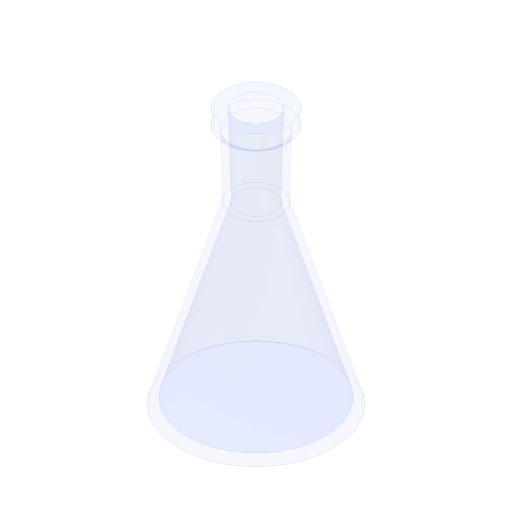
# Autodesk Inventor part: Модель колба коническая 25мл
Saved by Autodesk Inventor 2023 (Build 270158000, 158)
## iProperties
Created: 2022-06-09
Part Number: Модель колба коническая 25мл
Material: Типовые
Document SubType Name: Modeling
Designer: Admin
Density: 1 g/cm^3
Appearance: Вода — пузырьки
Author: Admin
Autodesk Inventor part; units mm, degrees
ref_plane "YZ Plane" through (0, 0, 0) normal (1, 0, 0) x (0, 1, 0)
ref_plane "XZ Plane" through (0, 0, 0) normal (0, 1, 0) x (-1, 0, 0)
ref_plane "XY Plane" through (0, 0, 0) normal (0, 0, 1) x (1, 0, 0)
sketch "Эскиз1" plane through (0, 0, 0) normal (0, 0, 1) x (1, 0, 0)
  line L0 (0, 0) -> (25.5, 0)
  line L1 (25.5, 0) -> (8, 58)
  line L2 (8, 58) -> (8.4582, 79)
  line L3 (10.5, 80) -> (10.5, 85)
  line L4 (10.5, 85) -> (6.5, 85)
  line L5 (6.5, 85) -> (5.9109, 58)
  line L6 (5.9109, 58) -> (22.8075, 2)
  line L7 (22.8075, 2) -> (0, 2)
  line L8 (0, 21.2466) -> (0, -2.9394)
  line L9 (8.4582, 79) -> (10.5, 80)
  line L10 (0, 0) -> (-25.5, 0)
  line L11 (-25.5, 0) -> (-8, 58)
  line L12 (-8, 58) -> (-8.4582, 79)
  line L13 (-10.5, 80) -> (-10.5, 85)
  line L14 (-10.5, 85) -> (-6.5, 85)
  line L15 (-6.5, 85) -> (-5.9109, 58)
  line L16 (-5.9109, 58) -> (-22.8075, 2)
  line L17 (-22.8075, 2) -> (0, 2)
  line L18 (-8.4582, 79) -> (-10.5, 80)
  line L19 (43.1283, 50) -> (10.4138, 50)
  line L20 (10.4138, 50) -> (8.3785, 49.8219)
  line L21 (-9.1205, 47.3626) -> (-11.1664, 47.5057)
  line L22 (-11.1664, 47.5057) -> (-43.7017, 44.0861)
  line L23 (25.1983, 1) -> (-25.1983, 1)
  line L24 (43.1283, -5) -> (-43.7017, -5)
  line L25 (-9.1205, 47.3626) -> (8.3785, 49.8219)
  point P0 (0, 2)
  dimension "d0" = 51
  dimension "d1" = 2
  dimension "d2" = 2
  dimension "d3" = 58
  dimension "d4" = 85
  dimension "d5" = 5
  dimension "d6" = 16
  dimension "d8" = 21
  dimension "d9" = 4
  dimension "d10" = 21
  dimension "d12" = 50
  dimension "d27" = 5
  dimension "d51" = 5
  dimension "d53" = 3
  dimension "d55" = 12
  dimension "d57" = 10
  dimension "d78" = 86.83
  constraints: 52 end point, 8 symmetric about line, 6 point on line, 4 parallel, 3 horizontal, 3 vertical alignment, 1 equal length, 1 horizontal alignment, 1 perpendicular, 1 vertical, 1 other
  measures "d0" diameter of L0.end L8
  measures "d1" distance between parallel lines of L7 L0
  measures "d2" distance between parallel lines of L1 L6
  measures "d3" vertical distance of L1.end L0.end
  measures "d4" distance between parallel lines of L4 L0
  measures "d5" distance of L3.start L3.end
  measures "d6" diameter of L1.end L8
  measures "d8" diameter of L3 L8
  measures "d9" distance of L3.end L4.end
  measures "d10" vertical distance of L2.end L1.end
  measures "d12" distance between parallel lines of L19 L0
  measures "d27" distance between parallel lines of L0 L24
  measures "d51" angle of L19 L20
  measures "d53" angle of L25 L20
  measures "d55" angle of L25 L21
  measures "d57" angle of L22 L21
  measures "d78" distance of L24.start L24.end
revolve "Вращение1" add sketch "Эскиз1" angle 360 about axis through (0, 21.2466, 0) along (0, -1, 0) contours L8 L23 L1 L0 | L8 L7 L6 L20 L1 L23 | L20 L6 L5 L4 L3 L9 L2 L1
ref_plane "РабПлоскость1" through (43.1283, 50, 0) normal (-1, 0, 0) x (0, -1, 0)
sketch "Эскиз2" plane through (43.1283, 50, 0) normal (-1, 0, 0) x (0, -1, 0)
  circle A0 centre (0, 0) radius 0.5
  point P0 (50, 0)
  dimension "d14" = 1
  constraints: 1 centre point, 1 coincident
  measures "d14" diameter of A0
sweep "Сдвиг1" add profiles "Эскиз2" path "Эскиз1" separate body path curves L19 L20 L25 L21 L22
ref_plane "РабПлоскость2" through (25.1983, 1, 0) normal (-1, 0, 0) x (0, -1, 0)
sketch "Эскиз3" plane through (25.1983, 1, 0) normal (-1, 0, 0) x (0, -1, 0)
  circle A0 centre (0, 0) radius 0.5
  point P0 (1, 0)
  dimension "d17" = 1
  constraints: 1 centre point, 1 coincident
  measures "d17" diameter of A0
ref_plane "РабПлоскость3" through (-25.1983, 1, 0) normal (-1, 0, 0) x (0, -1, 0)
sketch "Эскиз4" plane through (-25.1983, 1, 0) normal (-1, 0, 0) x (0, -1, 0)
  circle A0 centre (0, 0) radius 0.1
  point P0 (1, 0)
  dimension "d18" = 0.2
  constraints: 1 centre point, 1 coincident
  measures "d18" diameter of A0
loft "Лофт1" add profiles "Эскиз3", "Эскиз4" separate body
extrude "Выдавливание1" add sketch "Эскиз3" against normal up to surface (17.93 mm away) bodies 3
extrude "Выдавливание2" add sketch "Эскиз4" along normal blind 18.5 bodies 3
ref_plane "РабПлоскость4" through (43.1283, -5, 0) normal (-1, 0, 0) x (0, -1, 0)
sketch "Эскиз5" plane through (43.1283, -5, 0) normal (-1, 0, 0) x (0, -1, 0)
  circle A0 centre (0, 0) radius 0.5
  point P0 (-5, 0)
  dimension "d28" = 1
  constraints: 1 centre point, 1 coincident
  measures "d28" diameter of A0
sweep "Сдвиг2" add profiles "Эскиз5" path "Эскиз1" separate body path curves L24
sketch "Эскиз6" plane through (43.1283, 50, 0) normal (1, 0, 0) x (0, 0, -1)
  circle A0 centre (0, 0) radius 0.5 projected
  circle A1 centre (0, 0) radius 0.5 projected
  circle A2 centre (0, 0) radius 6
  circle A3 centre (0, -49) radius 0.5 projected
  circle A4 centre (0, -55) radius 0.5 projected
  circle A5 centre (0, -49) radius 2.5
  circle A6 centre (0, -55) radius 2.5
  point P0 (0, -50)
  dimension "d31" = 12
  dimension "d34" = 5
  dimension "d35" = 5
  constraints: 3 centre point, 3 coincident
  measures "d31" diameter of A2
  measures "d34" diameter of A5
  measures "d35" diameter of A6
extrude "Выдавливание3" add sketch "Эскиз6" along normal blind 50 separate body contours A0 | A2
extrude "Выдавливание4" add sketch "Эскиз6" along normal blind 10 contours A3 | A4 | A5 | A6 bodies 5
ref_plane "РабПлоскость5" through (-43.7017, 50, 0) normal (-1, 0, 0) x (0, 0, 1)
sketch "Эскиз9" plane through (-43.7017, 50, 0) normal (-1, 0, 0) x (0, 0, 1)
  circle A0 centre (0, -49) radius 0.5
  circle A1 centre (0, 0) radius 0.5
  circle A2 centre (0, 0) radius 1.5
  circle A3 centre (0, -49) radius 1.5
  circle A4 centre (0, -55) radius 0.5
  circle A5 centre (0, -55) radius 1.5
  circle A6 centre (0, 0) radius 0.5 projected
  circle A7 centre (0, -49) radius 0.5 projected
  circle A8 centre (0, -55) radius 0.5 projected
  circle A9 centre (0, -55) radius 0.5 projected
  circle A10 centre (0, -49) radius 1.5
  circle A11 centre (0, -55) radius 1.5
  circle A12 centre (0, 0) radius 1.5
  circle A13 centre (0, 1) radius 0.25
  circle A14 centre (0, -1) radius 0.25
  line L0 (0, 0) -> (0.8692, 0) construction
  circle A15 centre (0, -48) radius 0.25
  circle A16 centre (0, -50) radius 0.25
  line L1 (0, -49) -> (1.9722, -49) construction
  circle A17 centre (0, -54) radius 0.25
  circle A18 centre (0, -56) radius 0.25
  line L2 (0, -55) -> (2.8692, -55) construction
  point P0 (0, -48.4126)
  point P1 (0, -48.4126)
  point P2 (1, -49)
  dimension "d59" = 3
  dimension "d60" = 3
  dimension "d61" = 3
  dimension "d64" = 0.5
  dimension "d65" = 1
  dimension "d66" = 0.5
  dimension "d67" = 1
  dimension "d68" = 0.5
  dimension "d69" = 1
  constraints: 15 centre point, 10 coincident, 6 end point, 6 equal radius, 6 vertical alignment, 3 horizontal, 2 concentric, 3 other
  measures "d59" diameter of A2
  measures "d60" diameter of A3
  measures "d61" diameter of A5
  measures "d64" diameter of A13
  measures "d65" distance from line of L0 A13.centre
  measures "d66" diameter of A15
  measures "d67" distance from line of L1 A15.centre
  measures "d68" diameter of A17
  measures "d69" distance from line of L2 A17.centre
extrude "Выдавливание7" add sketch "Эскиз9" along normal blind 2 separate body contours A0 | A1 | A2 | A3 | A4 | A5 | A13 | A14 | A15 | A16 | A17 | A18
sketch "Эскиз10" plane through (-45.7017, 50, 0) normal (-1, 0, 0) x (0, 0, 1)
  circle A0 centre (0, -49) radius 1.5
  circle A1 centre (0, -55) radius 1.5
  circle A2 centre (0, 0) radius 1.5
  circle A3 centre (0, 1) radius 0.25
  circle A4 centre (0, -1) radius 0.25
  line L0 (0, 0) -> (0.8692, 0) construction
  circle A5 centre (0, -48) radius 0.25
  circle A6 centre (0, -50) radius 0.25
  line L1 (0, -49) -> (1.8692, -49) construction
  circle A7 centre (0, -54) radius 0.25
  circle A8 centre (0, -56) radius 0.25
  line L2 (0, -55) -> (2.8692, -55) construction
  circle A9 centre (0, 0) radius 1.5 projected
  circle A10 centre (0, -49) radius 1.5 projected
  circle A11 centre (0, -55) radius 1.5 projected
  point P0 (0, -50)
  point P1 (0, -48.4126)
  point P2 (1, -49)
  dimension "d70" = 0.5
  dimension "d71" = 1
  dimension "d72" = 0.5
  dimension "d73" = 1
  dimension "d74" = 0.5
  dimension "d75" = 1
  constraints: 9 centre point, 6 coincident, 6 end point, 6 equal radius, 6 vertical alignment, 3 horizontal, 3 other
  measures "d70" diameter of A3
  measures "d71" distance from line of L0 A3.centre
  measures "d72" diameter of A5
  measures "d73" distance from line of L1 A5.centre
  measures "d74" diameter of A7
  measures "d75" distance from line of L2 A7.centre
extrude "Выдавливание8" add sketch "Эскиз10" along normal blind 10 contours A3 | A4 | A5 | A6 | A7 | A8 bodies 6
